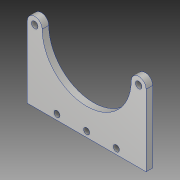
# Autodesk Inventor part: motor_end_plate
Saved by Autodesk Inventor 2019 (Build 230136000, 136)
## iProperties
Created: 2018-09-24
Part Number: motor_end_plate
Material: Aluminum 6061
Document SubType Name: Modeling
Designer: Callum Snowden
Mass: 72.2328 g
Surface Area: 119.007 cm^2
Volume: 26.7529 cm^3
Density: 2.7 g/cm^3
Appearance: Aluminum - Flat
Author: Callum Snowden
Autodesk Inventor part; units mm, degrees
ref_plane "YZ Plane" through (0, 0, 0) normal (1, 0, 0) x (0, 1, 0)
ref_plane "XZ Plane" through (0, 0, 0) normal (0, 1, 0) x (-1, 0, 0)
ref_plane "XY Plane" through (0, 0, 0) normal (0, 0, 1) x (1, 0, 0)
sketch "Sketch1" plane through (0, 0, 0) normal (0, 0, 1) x (1, 0, 0)
  line L0 (-75.6, 0) -> (75.6, 0) construction
  line L1 (0, 21.1) -> (0, -79.35) construction
  line L2 (54, 0) -> (54, -65)
  line L3 (54, -65) -> (-54, -65)
  line L4 (-54, -65) -> (-54, 0)
  circle A0 centre (47.25, 0) radius 3
  circle A1 centre (-47.25, 0) radius 3
  arc A2 (-40.5, 0) -> (-54, 0) centre (-47.25, 0) ccw
  arc A3 (54, 0) -> (40.5, 0) centre (47.25, 0) ccw
  arc A4 (-40.5, 0) -> (40.5, 0) centre (0, 0) ccw
  line L5 (-54, -60) -> (54, -60) construction
  circle A5 centre (0, -60) radius 2.75
  circle A6 centre (-27, -60) radius 2.75
  circle A7 centre (27, -60) radius 2.75
  dimension "d0" = 108
  dimension "d2" = 6
  dimension "d3" = 6
  dimension "d6" = 94.5
  dimension "d9" = 65
  dimension "d21" = 5
  dimension "d23" = 5.5
  dimension "d24" = 5.5
  dimension "d25" = 5.5
  dimension "d26" = 54
  constraints: 8 centre point, 8 end point, 6 point on circle, 6 point on line, 4 tangent, 2 coincident, 2 parallel, 2 symmetric about line, 1 line through centre, 1 midpoint, 1 perpendicular, 1 other
  measures "d0" distance of L2.end L3.end
  measures "d2" diameter of A0
  measures "d3" diameter of A1
  measures "d6" distance of A1.centre A0.centre
  measures "d9" distance of L3.end L4.end
  measures "d21" distance between parallel lines of L3 L5
  measures "d23" diameter of A5
  measures "d24" diameter of A6
  measures "d25" diameter of A7
  measures "d26" distance of A7.centre A6.centre
extrude "Extrusion2" add sketch "Sketch1" along normal blind 6
body "Solid2"
